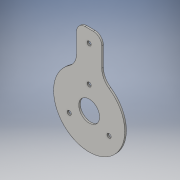
# Autodesk Inventor part: door_clamp
Saved by Autodesk Inventor 2016 (Build 200138000, 138)
## iProperties
Created: 2015-07-20
Part Number: door_clamp
Material: Generic
Document SubType Name: Modeling
Designer: chdsbd
Density: 1 g/cm^3
Appearance: Default
Author: chdsbd
Autodesk Inventor part; units mm, degrees
ref_plane "YZ Plane" through (0, 0, 0) normal (1, 0, 0) x (0, 1, 0)
ref_plane "XZ Plane" through (0, 0, 0) normal (0, 1, 0) x (-1, 0, 0)
ref_plane "XY Plane" through (0, 0, 0) normal (0, 0, 1) x (1, 0, 0)
sketch "Sketch1" plane through (0, 0, 0) normal (0, 0, 1) x (1, 0, 0)
  circle A0 centre (0, 0) radius 15.875
  arc A1 (-30.226, 44.7179) -> (30.226, 44.7179) centre (0, 0) ccw
  circle A2 centre (0, 0) radius 22.5683 construction
  circle A3 centre (0, 0) radius 34.925 construction
  circle A4 centre (0, 34.925) radius 3.175
  line L0 (0, 41.275) -> (0, 0) construction
  line L1 (-19.05, 65.7616) -> (-19.05, 95.25)
  line L2 (-6.35, 107.95) -> (6.35, 107.95)
  line L3 (19.05, 95.25) -> (19.05, 65.7616)
  line L4 (0, 0) -> (0, 107.95) construction
  circle A5 centre (0, 88.9) radius 3.175
  circle A6 centre (-30.2459, -17.4625) radius 3.175
  circle A7 centre (30.2459, -17.4625) radius 3.175
  arc A8 (-30.226, 44.7179) -> (-19.05, 65.7616) centre (-44.45, 65.7616) ccw
  arc A9 (19.05, 65.7616) -> (30.226, 44.7179) centre (44.45, 65.7616) ccw
  arc A10 (-6.35, 107.95) -> (-19.05, 95.25) centre (-6.35, 95.25) ccw
  arc A11 (19.05, 95.25) -> (6.35, 107.95) centre (6.35, 95.25) ccw
  point P0 (-19.05, 107.95)
  point P1 (19.05, 107.95)
  point P2 (19.05, 50.5015)
  point P3 (-19.05, 50.5015)
  dimension "d0" = 107.95
  dimension "d2" = 31.75
  dimension "d6" = 6.35
  dimension "d14" = 19.05
  dimension "d15" = 6.35
  dimension "d16" = 19.05
  dimension "d18" = 88.9
  dimension "d22" = 360
  dimension "d26" = 25.4
  dimension "d29" = 12.7
  dimension "d30" = 19.05
  constraints: 12 point on circle, 11 centre point, 10 end point, 9 point on line, 8 tangent, 4 coincident, 3 perpendicular, 2 equal radius, 2 vertical, 1 midpoint, 1 vertical alignment, 10 other
  measures "d0" diameter of A1
  measures "d2" diameter of A0
  measures "d6" diameter of A4
  measures "d14" distance between parallel lines of L4 L3
  measures "d15" diameter of A5
  measures "d16" distance from line of A5.centre L2
  measures "d18" distance of point (0, 0) A5.centre
  measures "d26" radius of A8
  measures "d29" radius of A10
extrude "Extrusion1" add sketch "Sketch1" along normal blind 2.54
body "Solid1"
